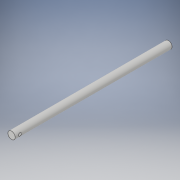
# Autodesk Inventor part: Hauptpfeiler
Saved by Autodesk Inventor 2019 (Build 230136000, 136)
## iProperties
Created: 2018-09-19
Part Number: Hauptpfeiler
Material: Generisch
Document SubType Name: Modeling
Designer: nico-
Density: 1 g/cm^3
Appearance: Vorgabe
Author: nico-
Autodesk Inventor part; units mm, degrees
ref_plane "YZ Plane" through (0, 0, 0) normal (1, 0, 0) x (0, 1, 0)
ref_plane "XZ Plane" through (0, 0, 0) normal (0, 1, 0) x (-1, 0, 0)
ref_plane "XY Plane" through (0, 0, 0) normal (0, 0, 1) x (1, 0, 0)
sketch "Skizze1" plane through (0, 0, 0) normal (0, 0, 1) x (1, 0, 0)
  circle A0 centre (0, 0) radius 7.5
  dimension "d0" = 15
  constraints: 1 centre point, 1 coincident
  measures "d0" diameter of A0
extrude "Extrusion1" add sketch "Skizze1" along normal mid plane 320
sketch "Skizze6" plane through (0, 0, 0) normal (1, 0, 0) x (0, 1, 0)
  circle A0 centre (0, 150) radius 3
  line L0 (-4.2, 0) -> (4.2, 0) projected
  point P0 (0, 0)
  dimension "d16" = 6
  dimension "d19" = 150
  constraints: 1 centre point
  measures "d16" diameter of A0
  measures "d19" distance from line of L0 A0.centre
extrude "Extrusion4" cut sketch "Skizze6" along normal mid plane 15
sketch "Skizze7" plane through (0, 0, -160) normal (0, 0, -1) x (-1, 0, 0)
  circle A0 centre (0, 0) radius 3
  dimension "d20" = 6
  constraints: 1 centre point, 1 coincident
  measures "d20" diameter of A0
extrude "Extrusion5" cut sketch "Skizze7" against normal blind 30
thread "Gewinde2" size "M6x1" class "6H" standard "ANSI Metric M Profile" full length
